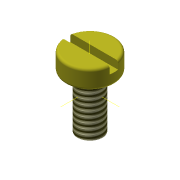
# Autodesk Inventor part: empty
Saved by Autodesk Inventor 2014 (Build 180170000, 170)
## iProperties
Created: 2015-04-13
Part Number: empty
Material: Generic
Document SubType Name: Modeling
Designer: Martin
Density: 1 g/cm^3
Appearance: Default
Author: Martin
Autodesk Inventor part; units mm, degrees
ref_plane "YZ Plane" through (0, 0, 0) normal (1, 0, 0) x (0, 1, 0)
ref_plane "XZ Plane" through (0, 0, 0) normal (0, 1, 0) x (-1, 0, 0)
ref_plane "XY Plane" through (0, 0, 0) normal (0, 0, 1) x (1, 0, 0)
sketch "Sketch1" plane through (0, 0, 0) normal (0, 1, 0) x (-1, 0, 0)
  line L0 (0, -3.815) -> (0, 3.815) projected
  line L1 (0, -2.725) -> (0, 2.725)
  line L2 (0, -2.725) -> (0.95, -2.725)
  line L3 (0.95, -2.725) -> (0.95, 1.275)
  line L4 (0.95, 1.275) -> (1.875, 1.275)
  line L5 (1.875, 1.275) -> (1.875, 2.725)
  line L6 (2.25, 0) -> (-0.375, 0) projected
  line L7 (0, 2.725) -> (1.875, 2.725)
  point P0 (0, 0)
  dimension "d0" = 4
  dimension "d1" = 1.9
  dimension "d3" = 3.75
  dimension "d4" = 1.45
  constraints: 12 end point, 4 perpendicular, 2 point on line, 1 parallel, 1 symmetric about line
  measures "d0" distance of L2.end L3.end
  measures "d1" diameter of L3 L0
  measures "d3" diameter of L5 L0
  measures "d4" distance of L4.end L5.end
revolve "Revolution1" add sketch "Sketch1" angle 360 about axis through (0, 0, -10) along (0, 0, 1)
thread "Thread2" size "M2x0.4" class "6g" standard "ANSI Metric M Profile" full length
fillet "Fillet1" radius 0.2 2 edges at (1.875, 0, 2.725) (1.875, 0, 1.275)
sketch "Sketch3" plane through (0, 0, 2.725) normal (0, 0, 1) x (1, 0, 0)
  circle A0 centre (0, 0) radius 1.875 projected
  circle A1 centre (0, 0) radius 1.875 projected
  line L0 (-2.5, -0.325) -> (2.5, -0.325)
  line L1 (2.5, -0.325) -> (2.5, 0.325)
  line L2 (2.5, 0.325) -> (-2.5, 0.325)
  line L3 (-2.5, 0.325) -> (-2.5, -0.325)
  line L4 (-2.5, -0.325) -> (2.5, 0.325) construction
  line L5 (2.5, -0.325) -> (-2.5, 0.325) construction
  dimension "d15" = 0.65
  dimension "d16" = 5
  constraints: 12 end point, 2 midpoint, 2 parallel, 1 horizontal, 1 perpendicular
  measures "d15" distance of L0.end L1.end
  measures "d16" distance of L1.end L2.end
extrude "Extrusion2" cut sketch "Sketch3" against normal blind 0.6 contours A0 L0 L2 | A0 L2 L1 L0 | A0 L0 L3 L2
body "Solid1"
